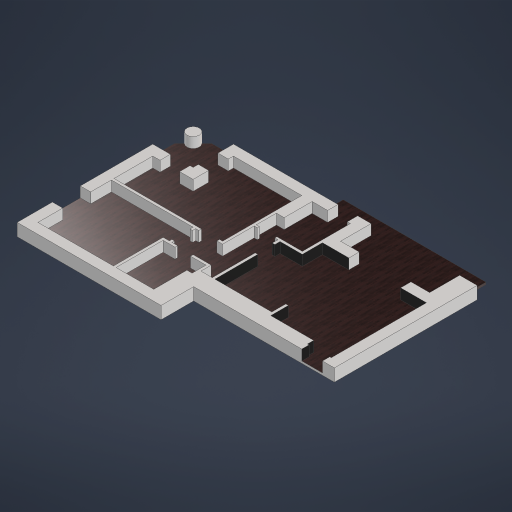
# Autodesk Inventor part: Torre nel Verde 17
Saved by Autodesk Inventor 2025.2 (Build 292293000, 293)
## iProperties
Created: 2025-08-11
Part Number: Torre nel Verde 17
Material: Generic
Document SubType Name: Modeling
Designer: Luca
Density: 1 g/cm^3
Appearance: Default
Mass: 7.02636e+07 g
Surface Area: 5.1785e+06 cm^2
Volume: 7.02636e+07 cm^3
Author: Luca
Autodesk Inventor part; units mm, degrees
ref_plane "YZ Plane" through (0, 0, 0) normal (1, 0, 0) x (0, 1, 0)
ref_plane "XZ Plane" through (0, 0, 0) normal (0, 1, 0) x (-1, 0, 0)
ref_plane "XY Plane" through (0, 0, 0) normal (0, 0, 1) x (1, 0, 0)
sketch "Sketch1" plane through (0, 0, 0) normal (0, 1, 0) x (-1, 0, 0)
  line L0 (0, 0) -> (-6950, 0)
  line L1 (-6950, 0) -> (-6950, -1575)
  line L2 (-13750, -1575) -> (-13750, -8475)
  line L3 (-13750, -8475) -> (-12900, -8475)
  line L4 (-12900, -8475) -> (-12900, -7025)
  line L5 (-12900, -7025) -> (-12000, -7025)
  line L6 (-12000, -7025) -> (-12000, -6525)
  line L7 (-12000, -6525) -> (-13250, -6525)
  line L8 (-13250, -6525) -> (-13250, -1925)
  line L9 (-13250, -1925) -> (-13175, -1925)
  line L10 (-13175, -1925) -> (-13175, -1575)
  line L11 (-12175, -1575) -> (-12175, -1925)
  line L12 (-12175, -1925) -> (-12100, -1925)
  line L13 (-12100, -1925) -> (-12100, -2225)
  line L14 (-12100, -2225) -> (-10025, -2225)
  line L15 (-10025, -2225) -> (-10025, -2400)
  line L16 (-10025, -2400) -> (-6350, -2400)
  line L17 (0, 0) -> (0, -1700)
  line L18 (0, -1700) -> (-500, -1700)
  line L19 (-500, -1700) -> (-500, -500)
  line L20 (-500, -500) -> (-6100, -500)
  line L21 (-6100, -500) -> (-6100, -2100)
  line L22 (-6100, -2100) -> (-6350, -2100)
  line L23 (-6350, -2100) -> (-6350, -2400)
  line L24 (0, -3050) -> (0, -6550)
  line L25 (0, -6550) -> (-850, -6550)
  line L26 (-850, -6550) -> (-850, -6050)
  line L27 (-850, -6050) -> (-500, -6050)
  line L28 (-500, -6050) -> (-500, -3050)
  line L29 (-500, -3050) -> (0, -3050)
  line L30 (-1800, -6550) -> (-1950, -6550)
  line L31 (-1950, -6550) -> (-1950, -6800)
  line L32 (-1950, -6800) -> (-2450, -6800)
  line L33 (-2450, -6800) -> (-2450, -6050)
  line L34 (-2450, -6050) -> (-1800, -6050)
  line L35 (-1800, -6050) -> (-1800, -6550)
  line L36 (-1950, -7750) -> (-2450, -7750)
  line L37 (-2450, -7750) -> (-2450, -8000)
  line L38 (-2450, -8000) -> (-5750, -8000)
  line L39 (-5750, -8000) -> (-5750, -6650)
  line L40 (-5750, -6650) -> (-6250, -6650)
  line L41 (-6250, -6650) -> (-6250, -8000)
  line L42 (-6250, -8000) -> (-7000, -8000)
  line L43 (-7000, -8000) -> (-7000, -8500)
  line L44 (-7000, -8500) -> (-1950, -8500)
  line L45 (-1950, -8500) -> (-1950, -7750)
  line L46 (-7950, -8500) -> (-7950, -8000)
  line L47 (-7950, -8000) -> (-8100, -8000)
  line L48 (-8100, -8000) -> (-8100, -6525)
  line L49 (-8100, -6525) -> (-9500, -6525)
  line L50 (-9500, -6525) -> (-9500, -7025)
  line L51 (-9500, -7025) -> (-8600, -7025)
  line L52 (-8600, -7025) -> (-8600, -8500)
  line L53 (-8600, -8500) -> (-7950, -8500)
  line L54 (-6950, -1575) -> (-12175, -1575)
  line L55 (-13175, -1575) -> (-13750, -1575)
  line L56 (-4275, -500) -> (-4275, -2775)
  line L57 (-4275, -2775) -> (-4850, -2775)
  line L58 (-4850, -2775) -> (-4850, -2900)
  line L59 (-4850, -2900) -> (-4575, -2900)
  line L60 (-4575, -2900) -> (-4575, -3025)
  line L61 (-4575, -3025) -> (-4450, -3025)
  line L62 (-4450, -3025) -> (-4450, -2900)
  line L63 (-4450, -2900) -> (-4150, -2900)
  line L64 (-4150, -2900) -> (-4150, -500)
  line L65 (-6350, -2400) -> (-6350, -2775)
  line L66 (-6350, -2775) -> (-5600, -2775)
  line L67 (-5600, -2775) -> (-5600, -2900)
  line L68 (-5600, -2900) -> (-6475, -2900)
  line L69 (-6475, -2900) -> (-6475, -2400)
  line L70 (-7025, -2400) -> (-7025, -4475)
  line L71 (-7025, -4475) -> (-7150, -4475)
  line L72 (-7150, -4475) -> (-7150, -2400)
  line L73 (-8100, -6525) -> (-8100, -5675)
  line L74 (-8100, -5675) -> (-6875, -5675)
  line L75 (-6875, -5675) -> (-6875, -5575)
  line L76 (-6875, -5575) -> (-7025, -5575)
  line L77 (-7025, -5575) -> (-7025, -5300)
  line L78 (-7025, -5300) -> (-7150, -5300)
  line L79 (-7150, -5300) -> (-7150, -5550)
  line L80 (-8225, -5550) -> (-8225, -6525)
  line L81 (-7150, -5550) -> (-8225, -5550)
  line L82 (-5875, -6650) -> (-5875, -5675)
  line L83 (-5875, -5675) -> (-6025, -5675)
  line L84 (-6025, -5675) -> (-6025, -5575)
  line L85 (-6025, -5575) -> (-5875, -5575)
  line L86 (-5875, -5575) -> (-5875, -4050)
  line L87 (-5875, -4050) -> (-5600, -4050)
  line L88 (-5600, -4050) -> (-5600, -4175)
  line L89 (-5600, -4175) -> (-5750, -4175)
  line L90 (-5750, -4175) -> (-5750, -6650)
  line L91 (-500, -4175) -> (-4725, -4175)
  line L92 (-4725, -4175) -> (-4725, -4050)
  line L93 (-4725, -4050) -> (-4575, -4050)
  line L94 (-4575, -4050) -> (-4575, -3900)
  line L95 (-4575, -3900) -> (-4450, -3900)
  line L96 (-4450, -3900) -> (-4450, -4050)
  line L97 (-4450, -4050) -> (-500, -4050)
  line L98 (-4150, -2900) -> (-4275, -2775) construction
  line L99 (-6350, -2775) -> (-6475, -2900) construction
  line L100 (-5750, -4175) -> (-5875, -4050) construction
  line L101 (0, -3050) -> (0, -1700)
  line L102 (-12175, -1575) -> (-13175, -1575)
  line L103 (-12000, -7025) -> (-9500, -7025)
  line L104 (-7000, -8500) -> (-7950, -8500)
  line L105 (0, -6550) -> (0, -7600)
  line L106 (-900, -8500) -> (-1950, -8500)
  circle A0 centre (-450, -8050) radius 300
  line L107 (0, -7600) -> (-237.868, -7837.868)
  line L108 (-662.132, -8262.132) -> (-900, -8500)
  line L109 (-850, -6050) -> (-1800, -6050)
  line L110 (-2450, -6800) -> (-2450, -7750)
  line L111 (-500, -3050) -> (-500, -1700)
  line L112 (-7000, -8000) -> (-7950, -8000)
  line L113 (-850, -6550) -> (-1800, -6550)
  line L114 (-1950, -6800) -> (-1950, -7750)
  line L115 (-9500, -6525) -> (-12000, -6525)
  line L116 (-6425, -8500) -> (-6425, -9325)
  line L117 (-6425, -9325) -> (-13325, -9325)
  line L118 (-13325, -9325) -> (-13325, -8475)
  line L119 (-13200, -8475) -> (-13200, -9200)
  line L120 (-13200, -9200) -> (-6550, -9200)
  line L121 (-6550, -9200) -> (-6550, -8500)
  line L122 (-6425, -9325) -> (-6550, -9200) construction
  line L123 (-13200, -9200) -> (-13325, -9325) construction
  line L124 (-7075, -9325) -> (-7075, -9200)
  line L125 (-8100, -5675) -> (-8225, -5550) construction
  line L126 (-10025, -2400) -> (-10025, -3075)
  line L127 (-10025, -3075) -> (-9900, -3075)
  line L128 (-9900, -3075) -> (-9900, -2400)
  dimension "d0" = 1000
  dimension "d1" = 3225
  dimension "d2" = 13250
  dimension "d4" = 1150
  dimension "d5" = 6075
  dimension "d6" = 5600
  dimension "d7" = 500
  dimension "d8" = 1350
  dimension "d9" = 1200
  dimension "d10" = 500
  dimension "d11" = 1600
  dimension "d12" = 1900
  dimension "d13" = 5850
  dimension "d14" = 6000
  dimension "d15" = 4300
  dimension "d16" = 6900
  dimension "d17" = 500
  dimension "d18" = 350
  dimension "d19" = 300
  dimension "d20" = 175
  dimension "d21" = 650
  dimension "d22" = 850
  dimension "d23" = 5550
  dimension "d24" = 5250
  dimension "d25" = 950
  dimension "d26" = 350
  dimension "d27" = 650
  dimension "d28" = 750
  dimension "d29" = 950
  dimension "d30" = 1950
  dimension "d31" = 1350
  dimension "d32" = 750
  dimension "d33" = 950
  dimension "d34" = 1850
  dimension "d35" = 500
  dimension "d36" = 2500
  dimension "d37" = 1400
  dimension "d38" = 900
  dimension "d41" = 875
  dimension "d42" = 1150
  dimension "d43" = 150
  dimension "d44" = 3950
  dimension "d45" = 3550
  dimension "d46" = 125
  dimension "d47" = 875
  dimension "d48" = 750
  dimension "d49" = 1500
  dimension "d52" = 3650
  dimension "d53" = 1825
  dimension "d57" = 600
  dimension "d58" = 1500
  dimension "d59" = 450
  dimension "d60" = 125
  dimension "d61" = 650
  dimension "d62" = 825
  dimension "d65" = 975
  dimension "d66" = 850
  dimension "d67" = 150
  dimension "d68" = 1150
  dimension "d69" = 825
  dimension "d70" = 250
  dimension "d71" = 275
  dimension "d72" = 100
  dimension "d73" = 125
  constraints: 259 end point, 95 perpendicular, 31 point on line, 21 collinear, 19 equal length, 12 vertical, 7 horizontal, 3 parallel, 2 point on circle, 1 centre point, 1 midpoint
  measures "d0" distance between parallel lines of L10 L11
  measures "d1" distance between parallel lines of L8 L15
  measures "d2" distance between parallel lines of L8 L17
  measures "d4" distance between parallel lines of L13 L8
  measures "d5" distance between parallel lines of L21 L11
  measures "d6" distance between parallel lines of L21 L19
  measures "d7" distance between parallel lines of L17 L19
  measures "d8" distance between parallel lines of L18 L29
  measures "d9" distance between parallel lines of L20 L18
  measures "d10" distance between parallel lines of L0 L20
  measures "d11" distance between parallel lines of L22 L20
  measures "d12" distance between parallel lines of L16 L20
  measures "d13" distance between parallel lines of L19 L23
  measures "d14" distance between parallel lines of L13 L21
  measures "d15" distance between parallel lines of L7 L14
  measures "d16" distance between parallel lines of L55 L3
  measures "d17" distance between parallel lines of L2 L8
  measures "d18" distance between parallel lines of L55 L9
  measures "d19" distance of L12.end L13.end
  measures "d20" distance between parallel lines of L14 L16
  measures "d21" distance between parallel lines of L14 L54
  measures "d22" distance between parallel lines of L1 L21
  measures "d23" distance between parallel lines of L20 L27
  measures "d24" distance between parallel lines of L39 L28
  measures "d25" distance between parallel lines of L35 L26
  measures "d26" distance between parallel lines of L26 L28
  measures "d27" distance between parallel lines of L33 L35
  measures "d28" distance between parallel lines of L34 L32
  measures "d29" distance between parallel lines of L32 L36
  measures "d30" distance between parallel lines of L34 L38
  measures "d31" distance between parallel lines of L40 L38
  measures "d32" distance between parallel lines of L43 L41
  measures "d33" distance between parallel lines of L46 L43
  measures "d34" distance between parallel lines of L48 L41
  measures "d35" distance between parallel lines of L52 L48
  measures "d36" distance between parallel lines of L6 L50
  measures "d37" distance between parallel lines of L50 L48
  measures "d38" distance between parallel lines of L6 L4
  measures "d41" distance between parallel lines of L61 L95
  measures "d42" distance between parallel lines of L63 L97
  measures "d43" distance between parallel lines of L95 L97
  measures "d44" distance between parallel lines of L96 L28
  measures "d45" distance between parallel lines of L20 L97
  measures "d46" distance between parallel lines of L91 L97
  measures "d47" distance between parallel lines of L88 L92
  measures "d48" distance between parallel lines of L67 L58
  measures "d49" distance between parallel lines of L58 L65
  measures "d52" distance between parallel lines of L19 L64
  measures "d53" distance between parallel lines of L21 L56
  measures "d57" diameter of A0
  measures "d58" distance from line of A0.centre L45
  measures "d59" distance between parallel lines of L43 L121
  measures "d60" distance between parallel lines of L121 L116
  measures "d61" distance between parallel lines of L124 L116
  measures "d62" distance between parallel lines of L44 L117
  measures "d65" distance between parallel lines of L83 L40
  measures "d66" distance between parallel lines of L75 L84
  measures "d67" distance between parallel lines of L82 L84
  measures "d68" distance between parallel lines of L77 L86
  measures "d69" distance between parallel lines of L71 L78
  measures "d70" distance between parallel lines of L81 L78
  measures "d71" distance between parallel lines of L78 L76
  measures "d72" distance between parallel lines of L74 L76
  measures "d73" distance between parallel lines of L81 L74
extrude "Extrusion1" add sketch "Sketch1" along normal blind 500 contours L17 L18 L19 L20 L21 L22 L23 L16 L15 L14 L13 L12 L11 L54 L1 L0 | L24 L25 L26 L27 L28 L29 | L10 L9 L8 L7 L6 L5 L4 L3 L2 L55 | L30 L31 L32 L33 L34 L35 | A0 | L45 L44 L43 L42 L41 L40 L39 L38 L37 L36 | L49 L48 L47 L46 L53 L52 L51 L50
extrude "Extrusion2" add sketch "Sketch1" along normal up to surface (500 mm away) contours L64 L63 L62 L61 L60 L59 L58 L57 L56 L20 | L28 L91 L92 L93 L94 L95 L96 L97 | L65 L66 L67 L68 L69 L16 | L16 L70 L71 L72 | L80 L81 L79 L78 L77 L76 L75 L74 L73 L49 | L40 L82 L83 L84 L85 L86 L87 L88 L89 L90
extrude "Extrusion3" add sketch "Sketch1" against normal blind 100
extrude "Extrusion4" add sketch "Sketch1" along normal up to surface (500 mm away) contours L16 L128 L127 L126
equation "\"d10\" = d7"
equation "\"d17\" = d10"
equation "\"d29\" = d25"
equation "\"d35\" = d7"
body "Solid1"
